Autodesk Fusion 360 part; units mm, degrees
(part 2 of 2)
sketch "Sketch4" plane through (0, 0, 14) normal (0, 0, 1) x (-1, 0, 0)
  circle A0 centre (0, 0) radius 13
  arc A1 (-1.2404, -19.3807) -> (-1.1473, -19.4662) centre (-1.1414, -19.3664) ccw
  arc A2 (-1.1473, -19.4662) -> (-0.8279, -19.4824) centre (0, 0) ccw
  arc A3 (-0.8279, -19.4824) -> (-0.7267, -19.4068) centre (-0.8237, -19.3825) ccw
  line L0 (-0.7267, -19.4068) -> (-0.5379, -18.6515)
  arc A4 (-0.3438, -18.5) -> (-0.5379, -18.6515) centre (-0.3438, -18.7) ccw
  line L1 (-0.3438, -18.5) -> (0.3438, -18.5)
  arc A5 (0.5379, -18.6515) -> (0.3438, -18.5) centre (0.3438, -18.7) ccw
  line L2 (0.5379, -18.6515) -> (0.7267, -19.4068)
  arc A6 (0.7267, -19.4068) -> (0.8279, -19.4824) centre (0.8237, -19.3825) ccw
  arc A7 (0.8279, -19.4824) -> (1.1473, -19.4662) centre (0, 0) ccw
  arc A8 (1.1473, -19.4662) -> (1.2404, -19.3807) centre (1.1414, -19.3664) ccw
  line L3 (1.2404, -19.3807) -> (1.3518, -18.6102)
  arc A9 (1.5295, -18.4399) -> (1.3518, -18.6102) centre (1.5498, -18.6388) ccw
  line L4 (1.5295, -18.4399) -> (2.2137, -18.3703)
  arc A10 (2.4221, -18.5014) -> (2.2137, -18.3703) centre (2.2339, -18.5693) ccw
  line L5 (2.4221, -18.5014) -> (2.6863, -19.2337)
  arc A11 (2.6863, -19.2337) -> (2.7947, -19.2987) centre (2.7804, -19.1997) ccw
  arc A12 (2.7947, -19.2987) -> (3.1108, -19.2503) centre (0, 0) ccw
  arc A13 (3.1108, -19.2503) -> (3.1947, -19.1558) centre (3.0948, -19.1516) ccw
  line L6 (3.1947, -19.1558) -> (3.2277, -18.378)
  arc A14 (3.3872, -18.1905) -> (3.2277, -18.378) centre (3.4275, -18.3864) ccw
  line L7 (3.3872, -18.1905) -> (4.0608, -18.0521)
  arc A15 (4.2814, -18.1614) -> (4.0608, -18.0521) centre (4.1011, -18.248) ccw
  line L8 (4.2814, -18.1614) -> (4.6184, -18.8632)
  arc A16 (4.6184, -18.8632) -> (4.7328, -18.9169) centre (4.7085, -18.8199) ccw
  arc A17 (4.7328, -18.9169) -> (5.0423, -18.8368) centre (0, 0) ccw
  arc A18 (5.0423, -18.8368) -> (5.1163, -18.7343) centre (5.0165, -18.7402) ccw
  line L9 (5.1163, -18.7343) -> (5.0704, -17.9571)
  arc A19 (5.2101, -17.7545) -> (5.0704, -17.9571) centre (5.27, -17.9453) ccw
  line L10 (5.2101, -17.7545) -> (5.8663, -17.5486)
  arc A20 (6.0968, -17.6351) -> (5.8663, -17.5486) centre (5.9262, -17.7395) ccw
  line L11 (6.0968, -17.6351) -> (6.503, -18.2992)
  arc A21 (6.503, -18.2992) -> (6.6223, -18.3411) centre (6.5883, -18.247) ccw
  arc A22 (6.6223, -18.3411) -> (6.9222, -18.23) centre (0, 0) ccw
  arc A23 (6.9222, -18.23) -> (6.9854, -18.1206) centre (6.8867, -18.1365) ccw
  line L12 (6.9854, -18.1206) -> (6.861, -17.352)
  arc A24 (6.9796, -17.1363) -> (6.861, -17.352) centre (7.0585, -17.3201) ccw
  line L13 (6.9796, -17.1363) -> (7.6116, -16.8651)
  arc A25 (7.8496, -16.9278) -> (7.6116, -16.8651) centre (7.6904, -17.0489) ccw
  line L14 (7.8496, -16.9278) -> (8.321, -17.5474)
  arc A26 (8.321, -17.5474) -> (8.4439, -17.577) centre (8.4006, -17.4869) ccw
  arc A27 (8.4439, -17.577) -> (8.7309, -17.4362) centre (0, 0) ccw
  arc A28 (8.7309, -17.4362) -> (8.7828, -17.3209) centre (8.6862, -17.3468) ccw
  line L15 (8.7828, -17.3209) -> (8.5813, -16.5689)
  arc A29 (8.6774, -16.3423) -> (8.5813, -16.5689) centre (8.7745, -16.5172) ccw
  line L16 (8.6774, -16.3423) -> (9.2787, -16.0085)
  arc A30 (9.5219, -16.0468) -> (9.2787, -16.0085) centre (9.3758, -16.1834) ccw
  line L17 (9.5219, -16.0468) -> (10.0535, -16.6156)
  arc A31 (10.0535, -16.6156) -> (10.1788, -16.6326) centre (10.1266, -16.5473) ccw
  arc A32 (10.1788, -16.6326) -> (10.4501, -16.4634) centre (0, 0) ccw
  arc A33 (10.4501, -16.4634) -> (10.49, -16.3435) centre (10.3965, -16.379) ccw
  line L18 (10.49, -16.3435) -> (10.2135, -15.6157)
  arc A34 (10.2862, -15.3806) -> (10.2135, -15.6157) centre (10.4005, -15.5447) ccw
  line L19 (10.2862, -15.3806) -> (10.8507, -14.9877)
  arc A35 (11.0965, -15.0012) -> (10.8507, -14.9877) centre (10.9649, -15.1518) ccw
  line L20 (11.0965, -15.0012) -> (11.6829, -15.5132)
  arc A36 (11.6829, -15.5132) -> (11.8092, -15.5175) centre (11.7487, -15.4379) ccw
  arc A37 (11.8092, -15.5175) -> (12.0621, -15.3217) centre (0, 0) ccw
  arc A38 (12.0621, -15.3217) -> (12.0896, -15.1984) centre (12.0002, -15.2432) ccw
  line L21 (12.0896, -15.1984) -> (11.741, -14.5023)
  arc A39 (11.7895, -14.261) -> (11.741, -14.5023) centre (11.9198, -14.4127) ccw
  line L22 (11.7895, -14.261) -> (12.3113, -13.8131)
  arc A40 (12.5572, -13.8016) -> (12.3113, -13.8131) centre (12.4416, -13.9648) ccw
  line L23 (12.5572, -13.8016) -> (13.1924, -14.2517)
  arc A41 (13.1924, -14.2517) -> (13.3185, -14.2431) centre (13.2502, -14.1701) ccw
  arc A42 (13.3185, -14.2431) -> (13.5503, -14.0228) centre (0, 0) ccw
  arc A43 (13.5503, -14.0228) -> (13.5652, -13.8973) centre (13.4808, -13.9509) ccw
  line L24 (13.5652, -13.8973) -> (13.1479, -13.2401)
  arc A44 (13.1718, -12.9951) -> (13.1479, -13.2401) centre (13.3167, -13.1329) ccw
  line L25 (13.1718, -12.9951) -> (13.6456, -12.4967)
  arc A45 (13.889, -12.4604) -> (13.6456, -12.4967) centre (13.7905, -12.6345) ccw
  line L26 (13.889, -12.4604) -> (14.5665, -12.8439)
  arc A46 (14.5665, -12.8439) -> (14.6911, -12.8226) centre (14.6158, -12.7569) ccw
  arc A47 (14.6911, -12.8226) -> (14.8994, -12.58) centre (0, 0) ccw
  arc A48 (14.8994, -12.58) -> (14.9016, -12.4536) centre (14.823, -12.5155) ccw
  line L27 (14.9016, -12.4536) -> (14.4199, -11.842)
  arc A49 (14.4189, -11.5959) -> (14.4199, -11.842) centre (14.577, -11.7183) ccw
  line L28 (14.4189, -11.5959) -> (14.8398, -11.0521)
  arc A50 (15.0784, -10.9914) -> (14.8398, -11.0521) centre (14.998, -11.1745) ccw
  line L29 (15.0784, -10.9914) -> (15.7912, -11.3043)
  arc A51 (15.7912, -11.3043) -> (15.913, -11.2706) centre (15.8314, -11.2128) ccw
  arc A52 (15.913, -11.2706) -> (16.0957, -11.0081) centre (0, 0) ccw
  arc A53 (16.0957, -11.0081) -> (16.085, -10.8822) centre (16.0131, -10.9517) ccw
  line L30 (16.085, -10.8822) -> (15.544, -10.3224)
  arc A54 (15.518, -10.0776) -> (15.544, -10.3224) centre (15.6878, -10.1834) ccw
  line L31 (15.518, -10.0776) -> (15.8818, -9.494)
  arc A55 (16.113, -9.4095) -> (15.8818, -9.494) centre (16.0515, -9.5998) ccw
  line L32 (16.113, -9.4095) -> (16.8538, -9.6488)
  arc A56 (16.8538, -9.6488) -> (16.9716, -9.6029) centre (16.8846, -9.5536) ccw
  arc A57 (16.9716, -9.6029) -> (17.1268, -9.3233) centre (0, 0) ccw
  arc A58 (17.1268, -9.3233) -> (17.1034, -9.199) centre (17.0389, -9.2755) ccw
  line L33 (17.1034, -9.199) -> (16.5085, -8.6969)
  arc A59 (16.458, -8.456) -> (16.5085, -8.6969) centre (16.6375, -8.5441) ccw
  line L34 (16.458, -8.456) -> (16.7608, -7.8386)
  arc A60 (16.9823, -7.7311) -> (16.7608, -7.8386) centre (16.9404, -7.9267) ccw
  line L35 (16.9823, -7.7311) -> (17.7435, -7.8942)
  arc A61 (17.7435, -7.8942) -> (17.856, -7.8366) centre (17.7645, -7.7964) ccw
  arc A62 (17.856, -7.8366) -> (17.9821, -7.5428) centre (0, 0) ccw
  arc A63 (17.9821, -7.5428) -> (17.9463, -7.4215) centre (17.8899, -7.5041) ccw
  line L36 (17.9463, -7.4215) -> (17.3037, -6.9822)
  arc A64 (17.229, -6.7476) -> (17.3037, -6.9822) centre (17.4165, -6.817) ccw
  line L37 (17.229, -6.7476) -> (17.4678, -6.1027)
  arc A65 (17.6773, -5.9734) -> (17.4678, -6.1027) centre (17.6554, -6.1722) ccw
  line L38 (17.6773, -5.9734) -> (18.4511, -6.0586)
  arc A66 (18.4511, -6.0586) -> (18.5572, -5.9899) centre (18.4621, -5.9592) ccw
  arc A67 (18.5572, -5.9899) -> (18.653, -5.6848) centre (0, 0) ccw
  arc A68 (18.653, -5.6848) -> (18.6051, -5.5678) centre (18.5573, -5.6557) ccw
  line L39 (18.6051, -5.5678) -> (17.9213, -5.1957)
  arc A69 (17.8232, -4.9699) -> (17.9213, -5.1957) centre (18.0169, -5.0201) ccw
  line L40 (17.8232, -4.9699) -> (17.9956, -4.3042)
  arc A70 (18.1909, -4.1543) -> (17.9956, -4.3042) centre (18.1892, -4.3543) ccw
  line L41 (18.1909, -4.1543) -> (18.9694, -4.1609)
  arc A71 (18.9694, -4.1609) -> (19.068, -4.0818) centre (18.9702, -4.0609) ccw
  arc A72 (19.068, -4.0818) -> (19.1324, -3.7686) centre (0, 0) ccw
  arc A73 (19.1324, -3.7686) -> (19.0729, -3.657) centre (19.0343, -3.7493) ccw
  line L42 (19.0729, -3.657) -> (18.355, -3.356)
  arc A74 (18.2346, -3.1413) -> (18.355, -3.356) centre (18.4323, -3.1716) ccw
  line L43 (18.2346, -3.1413) -> (18.3387, -2.4615)
  arc A75 (18.5179, -2.2927) -> (18.3387, -2.4615) centre (18.5364, -2.4918) ccw
  line L44 (18.5179, -2.2927) -> (19.293, -2.2204)
  arc A76 (19.293, -2.2204) -> (19.3831, -2.1318) centre (19.2837, -2.1208) ccw
  arc A77 (19.3831, -2.1318) -> (19.4155, -1.8137) centre (0, 0) ccw
  arc A78 (19.4155, -1.8137) -> (19.345, -1.7087) centre (19.3159, -1.8044) ccw
  line L45 (19.345, -1.7087) -> (18.6003, -1.4819)
  arc A79 (18.4588, -1.2804) -> (18.6003, -1.4819) centre (18.6586, -1.2905) ccw
  line L46 (18.4588, -1.2804) -> (18.4937, -0.5936)
  arc A80 (18.6548, -0.4075) -> (18.4937, -0.5936) centre (18.6934, -0.6037) ccw
  line L47 (18.6548, -0.4075) -> (19.4187, -0.2572)
  arc A81 (19.4187, -0.2572) -> (19.4993, -0.1599) centre (19.3993, -0.1591) ccw
  arc A82 (19.4993, -0.1599) -> (19.4993, 0.1599) centre (0, 0) ccw
  arc A83 (19.4993, 0.1599) -> (19.4187, 0.2572) centre (19.3993, 0.1591) ccw
  line L48 (19.4187, 0.2572) -> (18.6548, 0.4075)
  arc A84 (18.4937, 0.5936) -> (18.6548, 0.4075) centre (18.6934, 0.6037) ccw
  line L49 (18.4937, 0.5936) -> (18.4588, 1.2804)
  arc A85 (18.6003, 1.4819) -> (18.4588, 1.2804) centre (18.6586, 1.2905) ccw
  line L50 (18.6003, 1.4819) -> (19.345, 1.7087)
  arc A86 (19.345, 1.7087) -> (19.4155, 1.8137) centre (19.3159, 1.8044) ccw
  arc A87 (19.4155, 1.8137) -> (19.3831, 2.1318) centre (0, 0) ccw
  arc A88 (19.3831, 2.1318) -> (19.293, 2.2204) centre (19.2837, 2.1208) ccw
  line L51 (19.293, 2.2204) -> (18.5179, 2.2927)
  arc A89 (18.3387, 2.4615) -> (18.5179, 2.2927) centre (18.5364, 2.4918) ccw
  line L52 (18.3387, 2.4615) -> (18.2346, 3.1413)
  arc A90 (18.355, 3.356) -> (18.2346, 3.1413) centre (18.4323, 3.1716) ccw
  line L53 (18.355, 3.356) -> (19.0729, 3.657)
  arc A91 (19.0729, 3.657) -> (19.1324, 3.7686) centre (19.0343, 3.7493) ccw
  arc A92 (19.1324, 3.7686) -> (19.068, 4.0818) centre (0, 0) ccw
  arc A93 (19.068, 4.0818) -> (18.9694, 4.1609) centre (18.9702, 4.0609) ccw
  line L54 (18.9694, 4.1609) -> (18.1909, 4.1543)
  arc A94 (17.9956, 4.3042) -> (18.1909, 4.1543) centre (18.1892, 4.3543) ccw
  line L55 (17.9956, 4.3042) -> (17.8232, 4.9699)
  arc A95 (17.9213, 5.1957) -> (17.8232, 4.9699) centre (18.0169, 5.0201) ccw
  line L56 (17.9213, 5.1957) -> (18.6051, 5.5678)
  arc A96 (18.6051, 5.5678) -> (18.653, 5.6848) centre (18.5573, 5.6557) ccw
  arc A97 (18.653, 5.6848) -> (18.5572, 5.9899) centre (0, 0) ccw
  arc A98 (18.5572, 5.9899) -> (18.4511, 6.0586) centre (18.4621, 5.9592) ccw
  line L57 (18.4511, 6.0586) -> (17.6773, 5.9734)
  arc A99 (17.4678, 6.1027) -> (17.6773, 5.9734) centre (17.6554, 6.1722) ccw
  line L58 (17.4678, 6.1027) -> (17.229, 6.7476)
  arc A100 (17.3037, 6.9822) -> (17.229, 6.7476) centre (17.4165, 6.817) ccw
  line L59 (17.3037, 6.9822) -> (17.9463, 7.4215)
  arc A101 (17.9463, 7.4215) -> (17.9821, 7.5428) centre (17.8899, 7.5041) ccw
  arc A102 (17.9821, 7.5428) -> (17.856, 7.8366) centre (0, 0) ccw
  arc A103 (17.856, 7.8366) -> (17.7435, 7.8942) centre (17.7645, 7.7964) ccw
  line L60 (17.7435, 7.8942) -> (16.9823, 7.7311)
  arc A104 (16.7608, 7.8386) -> (16.9823, 7.7311) centre (16.9404, 7.9267) ccw
  line L61 (16.7608, 7.8386) -> (16.458, 8.456)
  arc A105 (16.5085, 8.6969) -> (16.458, 8.456) centre (16.6375, 8.5441) ccw
  line L62 (16.5085, 8.6969) -> (17.1034, 9.199)
  arc A106 (17.1034, 9.199) -> (17.1268, 9.3233) centre (17.0389, 9.2755) ccw
  arc A107 (17.1268, 9.3233) -> (16.9716, 9.6029) centre (0, 0) ccw
  arc A108 (16.9716, 9.6029) -> (16.8538, 9.6488) centre (16.8846, 9.5536) ccw
  line L63 (16.8538, 9.6488) -> (16.113, 9.4095)
  arc A109 (15.8818, 9.494) -> (16.113, 9.4095) centre (16.0515, 9.5998) ccw
  line L64 (15.8818, 9.494) -> (15.518, 10.0776)
  arc A110 (15.544, 10.3224) -> (15.518, 10.0776) centre (15.6878, 10.1834) ccw
  line L65 (15.544, 10.3224) -> (16.085, 10.8822)
  arc A111 (16.085, 10.8822) -> (16.0957, 11.0081) centre (16.0131, 10.9517) ccw
  arc A112 (16.0957, 11.0081) -> (15.913, 11.2706) centre (0, 0) ccw
  arc A113 (15.913, 11.2706) -> (15.7912, 11.3043) centre (15.8314, 11.2128) ccw
  line L66 (15.7912, 11.3043) -> (15.0784, 10.9914)
  arc A114 (14.8398, 11.0521) -> (15.0784, 10.9914) centre (14.998, 11.1745) ccw
  line L67 (14.8398, 11.0521) -> (14.4189, 11.5959)
  arc A115 (14.4199, 11.842) -> (14.4189, 11.5959) centre (14.577, 11.7183) ccw
  line L68 (14.4199, 11.842) -> (14.9016, 12.4536)
  arc A116 (14.9016, 12.4536) -> (14.8994, 12.58) centre (14.823, 12.5155) ccw
  arc A117 (14.8994, 12.58) -> (14.6911, 12.8226) centre (0, 0) ccw
  arc A118 (14.6911, 12.8226) -> (14.5665, 12.8439) centre (14.6158, 12.7569) ccw
  line L69 (14.5665, 12.8439) -> (13.889, 12.4604)
  arc A119 (13.6456, 12.4967) -> (13.889, 12.4604) centre (13.7905, 12.6345) ccw
  line L70 (13.6456, 12.4967) -> (13.1718, 12.9951)
  arc A120 (13.1479, 13.2401) -> (13.1718, 12.9951) centre (13.3167, 13.1329) ccw
  line L71 (13.1479, 13.2401) -> (13.5652, 13.8973)
  arc A121 (13.5652, 13.8973) -> (13.5503, 14.0228) centre (13.4808, 13.9509) ccw
  arc A122 (13.5503, 14.0228) -> (13.3185, 14.2431) centre (0, 0) ccw
  arc A123 (13.3185, 14.2431) -> (13.1924, 14.2517) centre (13.2502, 14.1701) ccw
  line L72 (13.1924, 14.2517) -> (12.5572, 13.8016)
  arc A124 (12.3113, 13.8131) -> (12.5572, 13.8016) centre (12.4416, 13.9648) ccw
  line L73 (12.3113, 13.8131) -> (11.7895, 14.261)
  arc A125 (11.741, 14.5023) -> (11.7895, 14.261) centre (11.9198, 14.4127) ccw
  line L74 (11.741, 14.5023) -> (12.0896, 15.1984)
  arc A126 (12.0896, 15.1984) -> (12.0621, 15.3217) centre (12.0002, 15.2432) ccw
  arc A127 (12.0621, 15.3217) -> (11.8092, 15.5175) centre (0, 0) ccw
  arc A128 (11.8092, 15.5175) -> (11.6829, 15.5132) centre (11.7487, 15.4379) ccw
  line L75 (11.6829, 15.5132) -> (11.0965, 15.0012)
  arc A129 (10.8507, 14.9877) -> (11.0965, 15.0012) centre (10.9649, 15.1518) ccw
  line L76 (10.8507, 14.9877) -> (10.2862, 15.3806)
  arc A130 (10.2135, 15.6157) -> (10.2862, 15.3806) centre (10.4005, 15.5447) ccw
  line L77 (10.2135, 15.6157) -> (10.49, 16.3435)
  arc A131 (10.49, 16.3435) -> (10.4501, 16.4634) centre (10.3965, 16.379) ccw
  arc A132 (10.4501, 16.4634) -> (10.1788, 16.6326) centre (0, 0) ccw
  arc A133 (10.1788, 16.6326) -> (10.0535, 16.6156) centre (10.1266, 16.5473) ccw
  line L78 (10.0535, 16.6156) -> (9.5219, 16.0468)
  arc A134 (9.2787, 16.0085) -> (9.5219, 16.0468) centre (9.3758, 16.1834) ccw
  line L79 (9.2787, 16.0085) -> (8.6774, 16.3423)
  arc A135 (8.5813, 16.5689) -> (8.6774, 16.3423) centre (8.7745, 16.5172) ccw
  line L80 (8.5813, 16.5689) -> (8.7828, 17.3209)
  arc A136 (8.7828, 17.3209) -> (8.7309, 17.4362) centre (8.6862, 17.3468) ccw
  arc A137 (8.7309, 17.4362) -> (8.4439, 17.577) centre (0, 0) ccw
  arc A138 (8.4439, 17.577) -> (8.321, 17.5474) centre (8.4006, 17.4869) ccw
  line L81 (8.321, 17.5474) -> (7.8496, 16.9278)
  arc A139 (7.6116, 16.8651) -> (7.8496, 16.9278) centre (7.6904, 17.0489) ccw
  line L82 (7.6116, 16.8651) -> (6.9796, 17.1363)
  arc A140 (6.861, 17.352) -> (6.9796, 17.1363) centre (7.0585, 17.3201) ccw
  line L83 (6.861, 17.352) -> (6.9854, 18.1206)
  arc A141 (6.9854, 18.1206) -> (6.9222, 18.23) centre (6.8867, 18.1365) ccw
  arc A142 (6.9222, 18.23) -> (6.6223, 18.3411) centre (0, 0) ccw
  arc A143 (6.6223, 18.3411) -> (6.503, 18.2992) centre (6.5883, 18.247) ccw
  line L84 (6.503, 18.2992) -> (6.0968, 17.6351)
  arc A144 (5.8663, 17.5486) -> (6.0968, 17.6351) centre (5.9262, 17.7395) ccw
  line L85 (5.8663, 17.5486) -> (5.2101, 17.7545)
  arc A145 (5.0704, 17.9571) -> (5.2101, 17.7545) centre (5.27, 17.9453) ccw
  line L86 (5.0704, 17.9571) -> (5.1163, 18.7343)
  arc A146 (5.1163, 18.7343) -> (5.0423, 18.8368) centre (5.0165, 18.7402) ccw
  arc A147 (5.0423, 18.8368) -> (4.7328, 18.9169) centre (0, 0) ccw
  arc A148 (4.7328, 18.9169) -> (4.6184, 18.8632) centre (4.7085, 18.8199) ccw
  line L87 (4.6184, 18.8632) -> (4.2814, 18.1614)
  arc A149 (4.0608, 18.0521) -> (4.2814, 18.1614) centre (4.1011, 18.248) ccw
  line L88 (4.0608, 18.0521) -> (3.3872, 18.1905)
  arc A150 (3.2277, 18.378) -> (3.3872, 18.1905) centre (3.4275, 18.3864) ccw
  line L89 (3.2277, 18.378) -> (3.1947, 19.1558)
  arc A151 (3.1947, 19.1558) -> (3.1108, 19.2503) centre (3.0948, 19.1516) ccw
  arc A152 (3.1108, 19.2503) -> (2.7947, 19.2987) centre (0, 0) ccw
  arc A153 (2.7947, 19.2987) -> (2.6863, 19.2337) centre (2.7804, 19.1997) ccw
  line L90 (2.6863, 19.2337) -> (2.4221, 18.5014)
  arc A154 (2.2137, 18.3703) -> (2.4221, 18.5014) centre (2.2339, 18.5693) ccw
  line L91 (2.2137, 18.3703) -> (1.5295, 18.4399)
  arc A155 (1.3518, 18.6102) -> (1.5295, 18.4399) centre (1.5498, 18.6388) ccw
  line L92 (1.3518, 18.6102) -> (1.2404, 19.3807)
  arc A156 (1.2404, 19.3807) -> (1.1473, 19.4662) centre (1.1414, 19.3664) ccw
  arc A157 (1.1473, 19.4662) -> (0.8279, 19.4824) centre (0, 0) ccw
  arc A158 (0.8279, 19.4824) -> (0.7267, 19.4068) centre (0.8237, 19.3825) ccw
  line L93 (0.7267, 19.4068) -> (0.5379, 18.6515)
  arc A159 (0.3438, 18.5) -> (0.5379, 18.6515) centre (0.3438, 18.7) ccw
  line L94 (0.3438, 18.5) -> (-0.3438, 18.5)
  arc A160 (-0.5379, 18.6515) -> (-0.3438, 18.5) centre (-0.3438, 18.7) ccw
  line L95 (-0.5379, 18.6515) -> (-0.7267, 19.4068)
  arc A161 (-0.7267, 19.4068) -> (-0.8279, 19.4824) centre (-0.8237, 19.3825) ccw
  arc A162 (-0.8279, 19.4824) -> (-1.1473, 19.4662) centre (0, 0) ccw
  arc A163 (-1.1473, 19.4662) -> (-1.2404, 19.3807) centre (-1.1414, 19.3664) ccw
  line L96 (-1.2404, 19.3807) -> (-1.3518, 18.6102)
  arc A164 (-1.5295, 18.4399) -> (-1.3518, 18.6102) centre (-1.5498, 18.6388) ccw
  line L97 (-1.5295, 18.4399) -> (-2.2137, 18.3703)
  arc A165 (-2.4221, 18.5014) -> (-2.2137, 18.3703) centre (-2.2339, 18.5693) ccw
  line L98 (-2.4221, 18.5014) -> (-2.6863, 19.2337)
  arc A166 (-2.6863, 19.2337) -> (-2.7947, 19.2987) centre (-2.7804, 19.1997) ccw
  arc A167 (-2.7947, 19.2987) -> (-3.1108, 19.2503) centre (0, 0) ccw
  arc A168 (-3.1108, 19.2503) -> (-3.1947, 19.1558) centre (-3.0948, 19.1516) ccw
  line L99 (-3.1947, 19.1558) -> (-3.2277, 18.378)
  arc A169 (-3.3872, 18.1905) -> (-3.2277, 18.378) centre (-3.4275, 18.3864) ccw
  line L100 (-3.3872, 18.1905) -> (-4.0608, 18.0521)
  arc A170 (-4.2814, 18.1614) -> (-4.0608, 18.0521) centre (-4.1011, 18.248) ccw
  line L101 (-4.2814, 18.1614) -> (-4.6184, 18.8632)
  arc A171 (-4.6184, 18.8632) -> (-4.7328, 18.9169) centre (-4.7085, 18.8199) ccw
  arc A172 (-4.7328, 18.9169) -> (-5.0423, 18.8368) centre (0, 0) ccw
  arc A173 (-5.0423, 18.8368) -> (-5.1163, 18.7343) centre (-5.0165, 18.7402) ccw
  line L102 (-5.1163, 18.7343) -> (-5.0704, 17.9571)
  arc A174 (-5.2101, 17.7545) -> (-5.0704, 17.9571) centre (-5.27, 17.9453) ccw
  line L103 (-5.2101, 17.7545) -> (-5.8663, 17.5486)
  arc A175 (-6.0968, 17.6351) -> (-5.8663, 17.5486) centre (-5.9262, 17.7395) ccw
  line L104 (-6.0968, 17.6351) -> (-6.503, 18.2992)
  arc A176 (-6.503, 18.2992) -> (-6.6223, 18.3411) centre (-6.5883, 18.247) ccw
  arc A177 (-6.6223, 18.3411) -> (-6.9222, 18.23) centre (0, 0) ccw
  arc A178 (-6.9222, 18.23) -> (-6.9854, 18.1206) centre (-6.8867, 18.1365) ccw
  line L105 (-6.9854, 18.1206) -> (-6.861, 17.352)
  arc A179 (-6.9796, 17.1363) -> (-6.861, 17.352) centre (-7.0585, 17.3201) ccw
  line L106 (-6.9796, 17.1363) -> (-7.6116, 16.8651)
  arc A180 (-7.8496, 16.9278) -> (-7.6116, 16.8651) centre (-7.6904, 17.0489) ccw
  line L107 (-7.8496, 16.9278) -> (-8.321, 17.5474)
  arc A181 (-8.321, 17.5474) -> (-8.4439, 17.577) centre (-8.4006, 17.4869) ccw
  arc A182 (-8.4439, 17.577) -> (-8.7309, 17.4362) centre (0, 0) ccw
  arc A183 (-8.7309, 17.4362) -> (-8.7828, 17.3209) centre (-8.6862, 17.3468) ccw
  line L108 (-8.7828, 17.3209) -> (-8.5813, 16.5689)
  arc A184 (-8.6774, 16.3423) -> (-8.5813, 16.5689) centre (-8.7745, 16.5172) ccw
  line L109 (-8.6774, 16.3423) -> (-9.2787, 16.0085)
  arc A185 (-9.5219, 16.0468) -> (-9.2787, 16.0085) centre (-9.3758, 16.1834) ccw
  line L110 (-9.5219, 16.0468) -> (-10.0535, 16.6156)
  arc A186 (-10.0535, 16.6156) -> (-10.1788, 16.6326) centre (-10.1266, 16.5473) ccw
  arc A187 (-10.1788, 16.6326) -> (-10.4501, 16.4634) centre (0, 0) ccw
  arc A188 (-10.4501, 16.4634) -> (-10.49, 16.3435) centre (-10.3965, 16.379) ccw
  line L111 (-10.49, 16.3435) -> (-10.2135, 15.6157)
  arc A189 (-10.2862, 15.3806) -> (-10.2135, 15.6157) centre (-10.4005, 15.5447) ccw
  line L112 (-10.2862, 15.3806) -> (-10.8507, 14.9877)
  arc A190 (-11.0965, 15.0012) -> (-10.8507, 14.9877) centre (-10.9649, 15.1518) ccw
  line L113 (-11.0965, 15.0012) -> (-11.6829, 15.5132)
  arc A191 (-11.6829, 15.5132) -> (-11.8092, 15.5175) centre (-11.7487, 15.4379) ccw
  arc A192 (-11.8092, 15.5175) -> (-12.0621, 15.3217) centre (0, 0) ccw
  arc A193 (-12.0621, 15.3217) -> (-12.0896, 15.1984) centre (-12.0002, 15.2432) ccw
  line L114 (-12.0896, 15.1984) -> (-11.741, 14.5023)
  arc A194 (-11.7895, 14.261) -> (-11.741, 14.5023) centre (-11.9198, 14.4127) ccw
  line L115 (-11.7895, 14.261) -> (-12.3113, 13.8131)
  arc A195 (-12.5572, 13.8016) -> (-12.3113, 13.8131) centre (-12.4416, 13.9648) ccw
  line L116 (-12.5572, 13.8016) -> (-13.1924, 14.2517)
  arc A196 (-13.1924, 14.2517) -> (-13.3185, 14.2431) centre (-13.2502, 14.1701) ccw
  arc A197 (-13.3185, 14.2431) -> (-13.5503, 14.0228) centre (0, 0) ccw
  arc A198 (-13.5503, 14.0228) -> (-13.5652, 13.8973) centre (-13.4808, 13.9509) ccw
  line L117 (-13.5652, 13.8973) -> (-13.1479, 13.2401)
  arc A199 (-13.1718, 12.9951) -> (-13.1479, 13.2401) centre (-13.3167, 13.1329) ccw
  line L118 (-13.1718, 12.9951) -> (-13.6456, 12.4967)
  arc A200 (-13.889, 12.4604) -> (-13.6456, 12.4967) centre (-13.7905, 12.6345) ccw
  line L119 (-13.889, 12.4604) -> (-14.5665, 12.8439)
  arc A201 (-14.5665, 12.8439) -> (-14.6911, 12.8226) centre (-14.6158, 12.7569) ccw
  arc A202 (-14.6911, 12.8226) -> (-14.8994, 12.58) centre (0, 0) ccw
  arc A203 (-14.8994, 12.58) -> (-14.9016, 12.4536) centre (-14.823, 12.5155) ccw
  line L120 (-14.9016, 12.4536) -> (-14.4199, 11.842)
  arc A204 (-14.4189, 11.5959) -> (-14.4199, 11.842) centre (-14.577, 11.7183) ccw
  line L121 (-14.4189, 11.5959) -> (-14.8398, 11.0521)
  arc A205 (-15.0784, 10.9914) -> (-14.8398, 11.0521) centre (-14.998, 11.1745) ccw
  line L122 (-15.0784, 10.9914) -> (-15.7912, 11.3043)
  arc A206 (-15.7912, 11.3043) -> (-15.913, 11.2706) centre (-15.8314, 11.2128) ccw
  arc A207 (-15.913, 11.2706) -> (-16.0957, 11.0081) centre (0, 0) ccw
  arc A208 (-16.0957, 11.0081) -> (-16.085, 10.8822) centre (-16.0131, 10.9517) ccw
  line L123 (-16.085, 10.8822) -> (-15.544, 10.3224)
  arc A209 (-15.518, 10.0776) -> (-15.544, 10.3224) centre (-15.6878, 10.1834) ccw
  line L124 (-15.518, 10.0776) -> (-15.8818, 9.494)
  arc A210 (-16.113, 9.4095) -> (-15.8818, 9.494) centre (-16.0515, 9.5998) ccw
  line L125 (-16.113, 9.4095) -> (-16.8538, 9.6488)
  arc A211 (-16.8538, 9.6488) -> (-16.9716, 9.6029) centre (-16.8846, 9.5536) ccw
  arc A212 (-16.9716, 9.6029) -> (-17.1268, 9.3233) centre (0, 0) ccw
  arc A213 (-17.1268, 9.3233) -> (-17.1034, 9.199) centre (-17.0389, 9.2755) ccw
  line L126 (-17.1034, 9.199) -> (-16.5085, 8.6969)
  arc A214 (-16.458, 8.456) -> (-16.5085, 8.6969) centre (-16.6375, 8.5441) ccw
  line L127 (-16.458, 8.456) -> (-16.7608, 7.8386)
  arc A215 (-16.9823, 7.7311) -> (-16.7608, 7.8386) centre (-16.9404, 7.9267) ccw
  line L128 (-16.9823, 7.7311) -> (-17.7435, 7.8942)
  arc A216 (-17.7435, 7.8942) -> (-17.856, 7.8366) centre (-17.7645, 7.7964) ccw
  arc A217 (-17.856, 7.8366) -> (-17.9821, 7.5428) centre (0, 0) ccw
  arc A218 (-17.9821, 7.5428) -> (-17.9463, 7.4215) centre (-17.8899, 7.5041) ccw
  line L129 (-17.9463, 7.4215) -> (-17.3037, 6.9822)
  arc A219 (-17.229, 6.7476) -> (-17.3037, 6.9822) centre (-17.4165, 6.817) ccw
  line L130 (-17.229, 6.7476) -> (-17.4678, 6.1027)
  arc A220 (-17.6773, 5.9734) -> (-17.4678, 6.1027) centre (-17.6554, 6.1722) ccw
  line L131 (-17.6773, 5.9734) -> (-18.4511, 6.0586)
  arc A221 (-18.4511, 6.0586) -> (-18.5572, 5.9899) centre (-18.4621, 5.9592) ccw
  arc A222 (-18.5572, 5.9899) -> (-18.653, 5.6848) centre (0, 0) ccw
  arc A223 (-18.653, 5.6848) -> (-18.6051, 5.5678) centre (-18.5573, 5.6557) ccw
  line L132 (-18.6051, 5.5678) -> (-17.9213, 5.1957)
  arc A224 (-17.8232, 4.9699) -> (-17.9213, 5.1957) centre (-18.0169, 5.0201) ccw
  line L133 (-17.8232, 4.9699) -> (-17.9956, 4.3042)
  arc A225 (-18.1909, 4.1543) -> (-17.9956, 4.3042) centre (-18.1892, 4.3543) ccw
  line L134 (-18.1909, 4.1543) -> (-18.9694, 4.1609)
  arc A226 (-18.9694, 4.1609) -> (-19.068, 4.0818) centre (-18.9702, 4.0609) ccw
  arc A227 (-19.068, 4.0818) -> (-19.1324, 3.7686) centre (0, 0) ccw
  arc A228 (-19.1324, 3.7686) -> (-19.0729, 3.657) centre (-19.0343, 3.7493) ccw
  line L135 (-19.0729, 3.657) -> (-18.355, 3.356)
  arc A229 (-18.2346, 3.1413) -> (-18.355, 3.356) centre (-18.4323, 3.1716) ccw
  line L136 (-18.2346, 3.1413) -> (-18.3387, 2.4615)
  arc A230 (-18.5179, 2.2927) -> (-18.3387, 2.4615) centre (-18.5364, 2.4918) ccw
  line L137 (-18.5179, 2.2927) -> (-19.293, 2.2204)
  arc A231 (-19.293, 2.2204) -> (-19.3831, 2.1318) centre (-19.2837, 2.1208) ccw
  arc A232 (-19.3831, 2.1318) -> (-19.4155, 1.8137) centre (0, 0) ccw
  arc A233 (-19.4155, 1.8137) -> (-19.345, 1.7087) centre (-19.3159, 1.8044) ccw
  line L138 (-19.345, 1.7087) -> (-18.6003, 1.4819)
  arc A234 (-18.4588, 1.2804) -> (-18.6003, 1.4819) centre (-18.6586, 1.2905) ccw
  line L139 (-18.4588, 1.2804) -> (-18.4937, 0.5936)
  arc A235 (-18.6548, 0.4075) -> (-18.4937, 0.5936) centre (-18.6934, 0.6037) ccw
  line L140 (-18.6548, 0.4075) -> (-19.4187, 0.2572)
  arc A236 (-19.4187, 0.2572) -> (-19.4993, 0.1599) centre (-19.3993, 0.1591) ccw
  arc A237 (-19.4993, 0.1599) -> (-19.4993, -0.1599) centre (0, 0) ccw
  arc A238 (-19.4993, -0.1599) -> (-19.4187, -0.2572) centre (-19.3993, -0.1591) ccw
  line L141 (-19.4187, -0.2572) -> (-18.6548, -0.4075)
  arc A239 (-18.4937, -0.5936) -> (-18.6548, -0.4075) centre (-18.6934, -0.6037) ccw
  line L142 (-18.4937, -0.5936) -> (-18.4588, -1.2804)
  arc A240 (-18.6003, -1.4819) -> (-18.4588, -1.2804) centre (-18.6586, -1.2905) ccw
  line L143 (-18.6003, -1.4819) -> (-19.345, -1.7087)
  arc A241 (-19.345, -1.7087) -> (-19.4155, -1.8137) centre (-19.3159, -1.8044) ccw
  arc A242 (-19.4155, -1.8137) -> (-19.3831, -2.1318) centre (0, 0) ccw
  arc A243 (-19.3831, -2.1318) -> (-19.293, -2.2204) centre (-19.2837, -2.1208) ccw
  line L144 (-19.293, -2.2204) -> (-18.5179, -2.2927)
  arc A244 (-18.3387, -2.4615) -> (-18.5179, -2.2927) centre (-18.5364, -2.4918) ccw
  line L145 (-18.3387, -2.4615) -> (-18.2346, -3.1413)
  arc A245 (-18.355, -3.356) -> (-18.2346, -3.1413) centre (-18.4323, -3.1716) ccw
  line L146 (-18.355, -3.356) -> (-19.0729, -3.657)
  arc A246 (-19.0729, -3.657) -> (-19.1324, -3.7686) centre (-19.0343, -3.7493) ccw
  arc A247 (-19.1324, -3.7686) -> (-19.068, -4.0818) centre (0, 0) ccw
  arc A248 (-19.068, -4.0818) -> (-18.9694, -4.1609) centre (-18.9702, -4.0609) ccw
  line L147 (-18.9694, -4.1609) -> (-18.1909, -4.1543)
  arc A249 (-17.9956, -4.3042) -> (-18.1909, -4.1543) centre (-18.1892, -4.3543) ccw
  line L148 (-17.9956, -4.3042) -> (-17.8232, -4.9699)
  arc A250 (-17.9213, -5.1957) -> (-17.8232, -4.9699) centre (-18.0169, -5.0201) ccw
  line L149 (-17.9213, -5.1957) -> (-18.6051, -5.5678)
  arc A251 (-18.6051, -5.5678) -> (-18.653, -5.6848) centre (-18.5573, -5.6557) ccw
  arc A252 (-18.653, -5.6848) -> (-18.5572, -5.9899) centre (0, 0) ccw
  arc A253 (-18.5572, -5.9899) -> (-18.4511, -6.0586) centre (-18.4621, -5.9592) ccw
  line L150 (-18.4511, -6.0586) -> (-17.6773, -5.9734)
  arc A254 (-17.4678, -6.1027) -> (-17.6773, -5.9734) centre (-17.6554, -6.1722) ccw
  line L151 (-17.4678, -6.1027) -> (-17.229, -6.7476)
  arc A255 (-17.3037, -6.9822) -> (-17.229, -6.7476) centre (-17.4165, -6.817) ccw
  line L152 (-17.3037, -6.9822) -> (-17.9463, -7.4215)
  arc A256 (-17.9463, -7.4215) -> (-17.9821, -7.5428) centre (-17.8899, -7.5041) ccw
  arc A257 (-17.9821, -7.5428) -> (-17.856, -7.8366) centre (0, 0) ccw
  arc A258 (-17.856, -7.8366) -> (-17.7435, -7.8942) centre (-17.7645, -7.7964) ccw
  line L153 (-17.7435, -7.8942) -> (-16.9823, -7.7311)
  arc A259 (-16.7608, -7.8386) -> (-16.9823, -7.7311) centre (-16.9404, -7.9267) ccw
  line L154 (-16.7608, -7.8386) -> (-16.458, -8.456)
  arc A260 (-16.5085, -8.6969) -> (-16.458, -8.456) centre (-16.6375, -8.5441) ccw
  line L155 (-16.5085, -8.6969) -> (-17.1034, -9.199)
  arc A261 (-17.1034, -9.199) -> (-17.1268, -9.3233) centre (-17.0389, -9.2755) ccw
  arc A262 (-17.1268, -9.3233) -> (-16.9716, -9.6029) centre (0, 0) ccw
  arc A263 (-16.9716, -9.6029) -> (-16.8538, -9.6488) centre (-16.8846, -9.5536) ccw
  line L156 (-16.8538, -9.6488) -> (-16.113, -9.4095)
  arc A264 (-15.8818, -9.494) -> (-16.113, -9.4095) centre (-16.0515, -9.5998) ccw
  line L157 (-15.8818, -9.494) -> (-15.518, -10.0776)
  arc A265 (-15.544, -10.3224) -> (-15.518, -10.0776) centre (-15.6878, -10.1834) ccw
  line L158 (-15.544, -10.3224) -> (-16.085, -10.8822)
  arc A266 (-16.085, -10.8822) -> (-16.0957, -11.0081) centre (-16.0131, -10.9517) ccw
  arc A267 (-16.0957, -11.0081) -> (-15.913, -11.2706) centre (0, 0) ccw
  arc A268 (-15.913, -11.2706) -> (-15.7912, -11.3043) centre (-15.8314, -11.2128) ccw
  line L159 (-15.7912, -11.3043) -> (-15.0784, -10.9914)
  arc A269 (-14.8398, -11.0521) -> (-15.0784, -10.9914) centre (-14.998, -11.1745) ccw
  line L160 (-14.8398, -11.0521) -> (-14.4189, -11.5959)
  arc A270 (-14.4199, -11.842) -> (-14.4189, -11.5959) centre (-14.577, -11.7183) ccw
  line L161 (-14.4199, -11.842) -> (-14.9016, -12.4536)
  arc A271 (-14.9016, -12.4536) -> (-14.8994, -12.58) centre (-14.823, -12.5155) ccw
  arc A272 (-14.8994, -12.58) -> (-14.6911, -12.8226) centre (0, 0) ccw
  arc A273 (-14.6911, -12.8226) -> (-14.5665, -12.8439) centre (-14.6158, -12.7569) ccw
  line L162 (-14.5665, -12.8439) -> (-13.889, -12.4604)
  arc A274 (-13.6456, -12.4967) -> (-13.889, -12.4604) centre (-13.7905, -12.6345) ccw
  line L163 (-13.6456, -12.4967) -> (-13.1718, -12.9951)
  arc A275 (-13.1479, -13.2401) -> (-13.1718, -12.9951) centre (-13.3167, -13.1329) ccw
  line L164 (-13.1479, -13.2401) -> (-13.5652, -13.8973)
  arc A276 (-13.5652, -13.8973) -> (-13.5503, -14.0228) centre (-13.4808, -13.9509) ccw
  arc A277 (-13.5503, -14.0228) -> (-13.3185, -14.2431) centre (0, 0) ccw
  arc A278 (-13.3185, -14.2431) -> (-13.1924, -14.2517) centre (-13.2502, -14.1701) ccw
  line L165 (-13.1924, -14.2517) -> (-12.5572, -13.8016)
  arc A279 (-12.3113, -13.8131) -> (-12.5572, -13.8016) centre (-12.4416, -13.9648) ccw
  line L166 (-12.3113, -13.8131) -> (-11.7895, -14.261)
  arc A280 (-11.741, -14.5023) -> (-11.7895, -14.261) centre (-11.9198, -14.4127) ccw
  line L167 (-11.741, -14.5023) -> (-12.0896, -15.1984)
  arc A281 (-12.0896, -15.1984) -> (-12.0621, -15.3217) centre (-12.0002, -15.2432) ccw
  arc A282 (-12.0621, -15.3217) -> (-11.8092, -15.5175) centre (0, 0) ccw
  arc A283 (-11.8092, -15.5175) -> (-11.6829, -15.5132) centre (-11.7487, -15.4379) ccw
  line L168 (-11.6829, -15.5132) -> (-11.0965, -15.0012)
  arc A284 (-10.8507, -14.9877) -> (-11.0965, -15.0012) centre (-10.9649, -15.1518) ccw
  line L169 (-10.8507, -14.9877) -> (-10.2862, -15.3806)
  arc A285 (-10.2135, -15.6157) -> (-10.2862, -15.3806) centre (-10.4005, -15.5447) ccw
  line L170 (-10.2135, -15.6157) -> (-10.49, -16.3435)
  arc A286 (-10.49, -16.3435) -> (-10.4501, -16.4634) centre (-10.3965, -16.379) ccw
  arc A287 (-10.4501, -16.4634) -> (-10.1788, -16.6326) centre (0, 0) ccw
  arc A288 (-10.1788, -16.6326) -> (-10.0535, -16.6156) centre (-10.1266, -16.5473) ccw
  line L171 (-10.0535, -16.6156) -> (-9.5219, -16.0468)
  arc A289 (-9.2787, -16.0085) -> (-9.5219, -16.0468) centre (-9.3758, -16.1834) ccw
  line L172 (-9.2787, -16.0085) -> (-8.6774, -16.3423)
  arc A290 (-8.5813, -16.5689) -> (-8.6774, -16.3423) centre (-8.7745, -16.5172) ccw
  line L173 (-8.5813, -16.5689) -> (-8.7828, -17.3209)
  arc A291 (-8.7828, -17.3209) -> (-8.7309, -17.4362) centre (-8.6862, -17.3468) ccw
  arc A292 (-8.7309, -17.4362) -> (-8.4439, -17.577) centre (0, 0) ccw
  arc A293 (-8.4439, -17.577) -> (-8.321, -17.5474) centre (-8.4006, -17.4869) ccw
  line L174 (-8.321, -17.5474) -> (-7.8496, -16.9278)
  arc A294 (-7.6116, -16.8651) -> (-7.8496, -16.9278) centre (-7.6904, -17.0489) ccw
  line L175 (-7.6116, -16.8651) -> (-6.9796, -17.1363)
  arc A295 (-6.861, -17.352) -> (-6.9796, -17.1363) centre (-7.0585, -17.3201) ccw
  line L176 (-6.861, -17.352) -> (-6.9854, -18.1206)
  arc A296 (-6.9854, -18.1206) -> (-6.9222, -18.23) centre (-6.8867, -18.1365) ccw
  arc A297 (-6.9222, -18.23) -> (-6.6223, -18.3411) centre (0, 0) ccw
  arc A298 (-6.6223, -18.3411) -> (-6.503, -18.2992) centre (-6.5883, -18.247) ccw
  line L177 (-6.503, -18.2992) -> (-6.0968, -17.6351)
  arc A299 (-5.8663, -17.5486) -> (-6.0968, -17.6351) centre (-5.9262, -17.7395) ccw
  line L178 (-5.8663, -17.5486) -> (-5.2101, -17.7545)
  arc A300 (-5.0704, -17.9571) -> (-5.2101, -17.7545) centre (-5.27, -17.9453) ccw
  line L179 (-5.0704, -17.9571) -> (-5.1163, -18.7343)
  arc A301 (-5.1163, -18.7343) -> (-5.0423, -18.8368) centre (-5.0165, -18.7402) ccw
  arc A302 (-5.0423, -18.8368) -> (-4.7328, -18.9169) centre (0, 0) ccw
  arc A303 (-4.7328, -18.9169) -> (-4.6184, -18.8632) centre (-4.7085, -18.8199) ccw
  line L180 (-4.6184, -18.8632) -> (-4.2814, -18.1614)
  arc A304 (-4.0608, -18.0521) -> (-4.2814, -18.1614) centre (-4.1011, -18.248) ccw
  line L181 (-4.0608, -18.0521) -> (-3.3872, -18.1905)
  arc A305 (-3.2277, -18.378) -> (-3.3872, -18.1905) centre (-3.4275, -18.3864) ccw
  line L182 (-3.2277, -18.378) -> (-3.1947, -19.1558)
  arc A306 (-3.1947, -19.1558) -> (-3.1108, -19.2503) centre (-3.0948, -19.1516) ccw
  arc A307 (-3.1108, -19.2503) -> (-2.7947, -19.2987) centre (0, 0) ccw
  arc A308 (-2.7947, -19.2987) -> (-2.6863, -19.2337) centre (-2.7804, -19.1997) ccw
  line L183 (-2.6863, -19.2337) -> (-2.4221, -18.5014)
  arc A309 (-2.2137, -18.3703) -> (-2.4221, -18.5014) centre (-2.2339, -18.5693) ccw
  line L184 (-2.2137, -18.3703) -> (-1.5295, -18.4399)
  arc A310 (-1.3518, -18.6102) -> (-1.5295, -18.4399) centre (-1.5498, -18.6388) ccw
  line L185 (-1.3518, -18.6102) -> (-1.2404, -19.3807)
  circle A311 centre (0, 0) radius 14
  dimension "d19" = 28
  constraint coincident A0.centre A2.centre
  measures "d19" diameter of A311
extrude "Extrude4" cut sketch "Sketch4" against normal blind 9 contours A311
